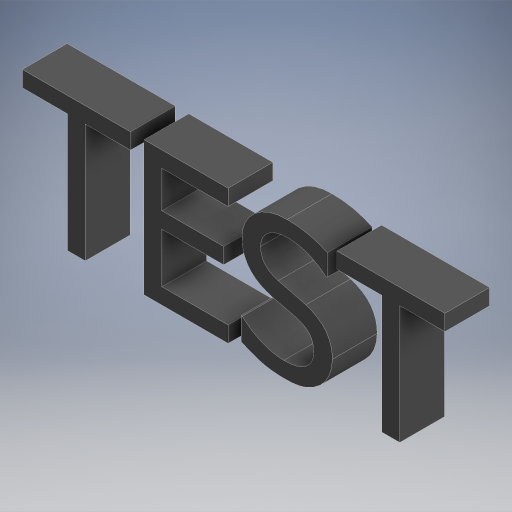
# Autodesk Inventor part: Standard - Amber select
Saved by Autodesk Inventor 2023 (Build 270158000, 158)
## iProperties
RuleStatus: InUse
Created: 2022-10-18
Part Number: Standard - Amber select
Material: Limestone
Document SubType Name: Modeling
Designer: awelt
Mass: 390.591 g
Surface Area: 451.209 cm^2
Volume: 150.227 cm^3
Density: 2.6 g/cm^3
Appearance: Generic
BoundingBL1: 1
BoundingBL2: 3 1/8
BoundingBL3: 9 7/16
Author: awelt
Autodesk Inventor part; units mm, degrees
ref_plane "YZ Plane" through (0, 0, 0) normal (1, 0, 0) x (0, 1, 0)
ref_plane "XZ Plane" through (0, 0, 0) normal (0, 1, 0) x (-1, 0, 0)
ref_plane "XY Plane" through (0, 0, 0) normal (0, 0, 1) x (1, 0, 0)
sketch "Sketch1" plane through (0, 0, 0) normal (0, 0, 1) x (1, 0, 0)
  line L0 (-0.0747, 67.8433) -> (64.3882, 67.8433) construction
  line L1 (64.3882, 67.8433) -> (64.3882, 0.2263) construction
  line L2 (64.3882, 0.2263) -> (-0.0747, 0.2263) construction
  line L3 (-0.0747, 0.2263) -> (-0.0747, 67.8433) construction
  line L4 (25.4282, -9.7152) -> (25.4282, 57.4693)
  line L5 (25.4282, 57.4693) -> (-0.1365, 57.4693)
  line L6 (-0.1365, 57.4693) -> (-0.1365, 66.4848)
  line L7 (-0.1365, 66.4848) -> (61.12, 66.4848)
  line L8 (61.12, 66.4848) -> (61.12, 57.4693)
  line L9 (61.12, 57.4693) -> (35.5553, 57.4693)
  line L10 (35.5553, 57.4693) -> (35.5553, -9.7152)
  line L11 (35.5553, -9.7152) -> (25.4282, -9.7152)
  line L12 (68.8388, -9.7152) -> (68.8388, 66.4848)
  line L13 (68.8388, 66.4848) -> (116.5101, 66.4848)
  line L14 (116.5101, 66.4848) -> (116.5101, 57.4693)
  line L15 (116.5101, 57.4693) -> (78.9658, 57.4693)
  line L16 (78.9658, 57.4693) -> (78.9658, 36.5976)
  line L17 (78.9658, 36.5976) -> (113.9783, 36.5976)
  line L18 (113.9783, 36.5976) -> (113.9783, 27.5821)
  line L19 (113.9783, 27.5821) -> (78.9658, 27.5821)
  line L20 (78.9658, 27.5821) -> (78.9658, -0.6996)
  line L21 (78.9658, -0.6996) -> (116.5101, -0.6996)
  line L22 (116.5101, -0.6996) -> (116.5101, -9.7152)
  line L23 (116.5101, -9.7152) -> (68.8388, -9.7152)
  spline S0 degree 2 poles (148.8673, -11.0737) (140.5927, -11.0737) (128.9836, -7.6156) (123.8584, -5.1456) knots 0 0 0 1 2 2 2
  line L24 (123.8584, -5.1456) -> (123.8584, 7.575)
  line L25 (123.8584, 7.575) -> (124.5994, 7.575)
  spline S1 degree 2 poles (124.5994, 7.575) (129.6011, 2.8819) (142.26, -2.3051) (148.1263, -2.3051) knots 0 0 0 1 2 2 2
  spline S2 degree 2 poles (148.1263, -2.3051) (156.5243, -2.3051) (165.1076, 4.6727) (165.1076, 10.4155) knots 0 0 0 1 2 2 2
  spline S3 degree 2 poles (165.1076, 10.4155) (165.1076, 14.985) (160.5999, 20.666) (155.7216, 22.0863) knots 0 0 0 1 2 2 2
  spline S4 degree 2 poles (155.7216, 22.0863) (152.2018, 23.0743) (146.3355, 24.4328) (141.9512, 25.5443) knots 0 0 0 1 2 2 2
  spline S5 degree 2 poles (141.9512, 25.5443) (137.9992, 26.5941) (131.7624, 29.7433) (129.3541, 32.2751) knots 0 0 0 1 2 2 2
  spline S6 degree 2 poles (129.3541, 32.2751) (127.0076, 34.8069) (124.4141, 41.5994) (124.4141, 46.0455) knots 0 0 0 1 2 2 2
  spline S7 degree 2 poles (124.4141, 46.0455) (124.4141, 55.308) (138.8637, 67.8433) (150.0405, 67.8433) knots 0 0 0 1 2 2 2
  spline S8 degree 2 poles (150.0405, 67.8433) (156.4626, 67.8433) (167.8246, 65.3116) (172.7029, 62.9033) knots 0 0 0 1 2 2 2
  line L26 (172.7029, 62.9033) -> (172.7029, 50.8002)
  line L27 (172.7029, 50.8002) -> (171.9619, 50.8002)
  spline S9 degree 2 poles (171.9619, 50.8002) (168.3187, 54.1348) (156.9566, 59.0748) (150.7198, 59.0748) knots 0 0 0 1 2 2 2
  spline S10 degree 2 poles (150.7198, 59.0748) (143.6802, 59.0748) (134.9734, 52.4675) (134.9734, 47.0952) knots 0 0 0 1 2 2 2
  spline S11 degree 2 poles (134.9734, 47.0952) (134.9734, 42.2787) (140.0987, 36.5359) (144.9152, 35.2391) knots 0 0 0 1 2 2 2
  spline S12 degree 2 poles (144.9152, 35.2391) (148.1263, 34.3746) (157.4506, 32.1516) (160.5381, 31.2254) knots 0 0 0 1 2 2 2
  spline S13 degree 2 poles (160.5381, 31.2254) (168.3804, 28.8171) (175.667, 19.1223) (175.667, 12.021) knots 0 0 0 1 2 2 2
  spline S14 degree 2 poles (175.667, 12.021) (175.667, 7.5132) (172.0237, -1.1319) (168.7509, -4.1576) knots 0 0 0 1 2 2 2
  spline S15 degree 2 poles (168.7509, -4.1576) (165.1076, -7.4921) (155.8451, -11.0737) (148.8673, -11.0737) knots 0 0 0 1 2 2 2
  line L28 (203.7634, -9.7152) -> (203.7634, 57.4693)
  line L29 (203.7634, 57.4693) -> (178.1987, 57.4693)
  line L30 (178.1987, 57.4693) -> (178.1987, 66.4848)
  line L31 (178.1987, 66.4848) -> (239.4551, 66.4848)
  line L32 (239.4551, 66.4848) -> (239.4551, 57.4693)
  line L33 (239.4551, 57.4693) -> (213.8905, 57.4693)
  line L34 (213.8905, 57.4693) -> (213.8905, -9.7152)
  line L35 (213.8905, -9.7152) -> (203.7634, -9.7152)
  point P0 (0, 0)
  constraints: 2 other
extrude "Extrusion1" add sketch "Sketch1" along normal blind 25.4
body "Solid1"
